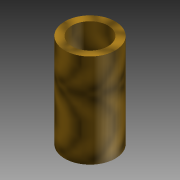
# Autodesk Inventor part: 13_0204_018
Saved by Autodesk Inventor 2012 SP1 (Build 160190100, 190)
## iProperties
GlobalPropertyList: <PropertyList/>
Created: 2013-03-28
Part Number: 13_0204_018
Material: Default
Document SubType Name: Modeling
Designer: vogel
Density: 1 g/cm^3
Author: vogel
Autodesk Inventor part; units mm, degrees
ref_plane "YZ Plane" through (0, 0, 0) normal (1, 0, 0) x (0, 1, 0)
ref_plane "XZ Plane" through (0, 0, 0) normal (0, 1, 0) x (-1, 0, 0)
ref_plane "XY Plane" through (0, 0, 0) normal (0, 0, 1) x (1, 0, 0)
sketch "Skizze1" plane through (0, 0, 0) normal (0, 0, 1) x (1, 0, 0)
  circle A0 centre (0, 0) radius 2.5
  circle A1 centre (0, 0) radius 3.5
  dimension "d0" = 7
  dimension "d1" = 5
  constraints: 2 centre point, 2 coincident
  measures "d0" diameter of A1
  measures "d1" diameter of A0
extrude "Extrusion1" add sketch "Skizze1" along normal blind 13
